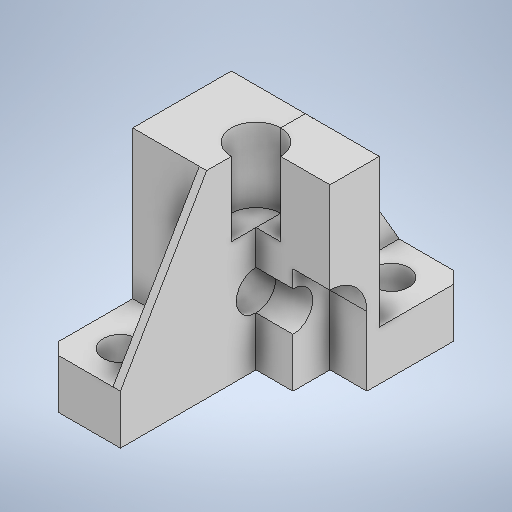
# Autodesk Inventor part: Деталь3
Saved by Autodesk Inventor 2025 (Build 290162000, 162)
## iProperties
Created: 2024-11-24
Part Number: Деталь3
Material: Типовые
Document SubType Name: Modeling
Designer: shoptick
Density: 1 g/cm^3
Appearance: По умолчанию
Author: shoptick
Autodesk Inventor part; units mm, degrees
ref_plane "YZ Plane" through (0, 0, 0) normal (1, 0, 0) x (0, 1, 0)
ref_plane "XZ Plane" through (0, 0, 0) normal (0, 1, 0) x (-1, 0, 0)
ref_plane "XY Plane" through (0, 0, 0) normal (0, 0, 1) x (1, 0, 0)
sketch "Эскиз1" plane through (0, 0, 0) normal (0, 1, 0) x (-1, 0, 0)
  line L0 (0, 0) -> (0, 55)
  line L1 (0, 55) -> (25, 55)
  line L2 (30, 0) -> (0, 0)
  line L3 (30, 50) -> (25, 55)
  line L4 (30, 50) -> (30, 0)
  circle A0 centre (15, 40) radius 7
  dimension "d0" = 55
  dimension "d6" = 14
  constraints: 10 end point, 2 vertical, 1 centre point, 1 perpendicular
  measures "d0" distance of L0.start L0.end
  measures "d6" diameter of A0
extrude "Выдавливание1" add sketch "Эскиз1" along normal blind 20
mirror "Зеркальное отражение1" about plane through (0, 0, 0) normal (0, 0, 1) of "Выдавливание1"
mirror "Зеркальное отражение2" about plane through (0, 0, 0) normal (1, 0, 0) of "Выдавливание1", "Зеркальное отражение1"
sketch "Эскиз2" plane through (0, 20, 0) normal (0, 1, 0) x (1, 0, 0)
  line L0 (-30, -50) -> (-30, 50) projected
  line L1 (-30, 0) -> (-30, -20)
  line L2 (-30, -20) -> (30, -20)
  line L3 (30, -20) -> (30, 20)
  line L4 (30, 20) -> (-30, 20)
  line L5 (-30, 20) -> (-30, 0)
  line L6 (-25, -55) -> (25, -55) projected
  line L7 (0, -55) -> (-3, -55)
  line L8 (-3, -55) -> (-3, -20)
  line L9 (0, -55) -> (3, -55)
  line L10 (3, -55) -> (3, -20)
  line L11 (25, 55) -> (-25, 55) projected
  line L12 (-3, 55) -> (-3, 20)
  line L13 (3, 20) -> (3, 55)
  point P0 (0, 0)
  dimension "d9" = 20
  dimension "d10" = 60
  dimension "d11" = 40
  dimension "d12" = 60
  dimension "d13" = 3
  dimension "d14" = 3
  constraints: 22 end point, 10 point on line, 5 perpendicular, 2 midpoint, 1 parallel, 1 vertical
  measures "d9" distance of L1.start L1.end
  measures "d10" distance of L1.end L2.end
  measures "d11" distance of L2.end L3.end
  measures "d12" distance of L3.end L4.end
  measures "d13" distance of L7.start L7.end
  measures "d14" distance of L7.start L9.end
extrude "Выдавливание2" add sketch "Эскиз2" along normal blind 60
sketch "Эскиз3" plane through (3, 20, 55) normal (1, 0, 0) x (0, 0, -1)
  line L0 (35, 60) -> (75, 60) projected
  line L1 (0, -20) -> (0, 0) projected
  line L2 (35, 60) -> (0, 0)
  line L3 (0, 0) -> (0, 60)
  line L4 (35, 60) -> (0, 60)
  line L5 (75, 0) -> (75, 60) projected
  line L6 (75, 60) -> (110.1116, 0)
  line L7 (110.1116, 0) -> (110.1116, 60)
  line L8 (110.1116, 60) -> (75, 60)
  point P0 (55, -20)
  constraints: 12 end point, 3 perpendicular, 1 collinear, 1 point on line
extrude "Выдавливание3" cut sketch "Эскиз3" against normal blind 60
sketch "Эскиз4" plane through (0, 80, 0) normal (0, 1, 0) x (1, 0, 0)
  circle A0 centre (0, 0) radius 10
  dimension "d19" = 20
  constraints: 1 centre point, 1 coincident
  measures "d19" diameter of A0
extrude "Выдавливание4" cut sketch "Эскиз4" against normal blind 30
sketch "Эскиз5" plane through (30, 0, 50) normal (1, 0, 0) x (0, 0, -1)
  line L0 (50, 0) -> (35, 0)
  line L1 (100, 0) -> (0, 0) projected
  line L2 (50, 0) -> (65, 0)
  line L3 (65, 0) -> (65, 28)
  line L4 (35, 0) -> (35, 28)
  arc A0 (65, 28) -> (35, 28) centre (50, 28) ccw
  dimension "d22" = 15
  dimension "d23" = 15
  dimension "d24" = 28
  dimension "d25" = 28
  dimension "d27" = 30
  constraints: 8 end point, 2 point on circle, 2 point on line, 1 centre point, 1 parallel, 1 perpendicular
  measures "d22" distance of L0.start L0.end
  measures "d23" distance of L0.start L2.end
  measures "d24" distance of L2.end L3.end
  measures "d25" distance of L4.end L0.end
  measures "d27" diameter of A0
extrude "Выдавливание5" cut sketch "Эскиз5" against normal blind 15
sketch "Эскиз6" plane through (15, 0, 50) normal (1, 0, 0) x (0, 0, -1)
  circle A0 centre (50, 28) radius 8
  point P0 (50, 0)
  dimension "d30" = 16
  constraints: 1 centre point
  measures "d30" diameter of A0
extrude "Выдавливание6" cut sketch "Эскиз6" against normal blind 60
sketch "Эскиз7" plane through (-30, 0, 50) normal (-1, 0, 0) x (0, 0, 1)
  line L0 (-65, 0) -> (-35, 0) projected
  line L1 (-65, 28) -> (-65, 0) projected
  line L2 (-65, 0) -> (-65, 28)
  line L3 (-35, 0) -> (-35, 28) projected
  line L4 (-35, 0) -> (-35, 28)
  arc A0 (-35, 28) -> (-65, 28) centre (-50, 28) ccw
  point P0 (-50, 0)
  dimension "d33" = 30
  constraints: 4 end point, 2 point on circle, 1 centre point, 1 collinear, 1 vertical
  measures "d33" diameter of A0
extrude "Выдавливание7" cut sketch "Эскиз7" against normal blind 15
split body "Разделение1" result two bodies by plane through (0, 0, 0) normal (1, 0, 0) first body at (0.5, 6.6861, -0.3214)
split "Разделение2" plane through (0, 0, 0) removes the side toward (0, 0, 1) bodies 2
